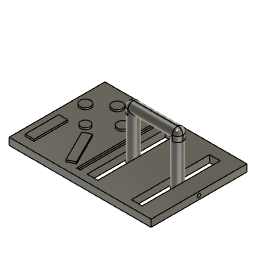
hardware final cad (Autodesk Fusion 360 design; units mm, degrees)
Autodesk Fusion 360 part; units mm, degrees
sketch "Sketch1" plane through (0, 0, 0) normal (0, 0, 1) x (1, 0, 0)
  line L0 (-8, -1) -> (1.5, -1)
  line L1 (1.5, -1) -> (1.5, -3.5)
  line L2 (1.5, -3.5) -> (-8, -3.5)
  line L3 (-8, -3.5) -> (-8, -1)
  line L4 (-11, 8) -> (-8, 8)
  line L5 (-8, 8) -> (-8, -14)
  line L6 (-8, -14) -> (-11, -14)
  line L7 (-11, -14) -> (-11, 8)
  line L8 (1.5, 8) -> (4.5, 8)
  line L9 (4.5, 8) -> (4.5, -14)
  line L10 (4.5, -14) -> (1.5, -14)
  line L11 (1.5, -14) -> (1.5, 8)
  line L12 (-19.5, -4) -> (-15, -13)
  line L13 (-15, -13) -> (-17, -14)
  line L14 (-17, -14) -> (-21.4999, -5.0003)
  line L15 (-19.5, -4) -> (-21.4999, -5.0003)
  line L16 (-29, -4) -> (-26.5, -4)
  line L17 (-26.5, -4) -> (-26.5, -13.5)
  line L18 (-26.5, -13.5) -> (-29, -13.5)
  line L19 (-29, -13.5) -> (-29, -4)
  circle A0 centre (-23, 6.5) radius 1.5
  circle A1 centre (-28, 2.5) radius 1.5
  circle A2 centre (-23, -2.5) radius 1.3194
  circle A3 centre (-17.5, 2.5) radius 1.5
  dimension "d1" = 10.062
  constraint horizontal L0
  constraint vertical L1
  constraint horizontal L2
  constraint vertical L3
  constraint horizontal L4
  constraint vertical L5
  constraint horizontal L6
  constraint vertical L7
  constraint horizontal L8
  constraint vertical L9
  constraint horizontal L10
  constraint vertical L11
  constraint perpendicular L12 L13
  constraint perpendicular L13 L14
  constraint horizontal L16
  constraint vertical L17
  constraint horizontal L18
  constraint vertical L19
  measures "d1" distance of L13.end L14.end
extrude "Extrude1" add sketch "Sketch1" along normal blind 1 makes body 1 at (-18.6666, -7.3334, 0) makes body 2 at (-23.2291, -1.2007, 0.6667) makes body 3 at (-16.0019, 2.4252, 0.6667) makes body 4 at (-28.1667, -7.1667, 0) makes body 5 at (-26.5019, 2.4252, 0.6667) makes body 6 at (-21.5019, 6.4252, 0.6667) makes body 7 at (-10, -3.1667, 0)
sketch "Sketch2" plane through (0, 0, 0) normal (0, 0, 1) x (1, 0, 0)
  line L0 (-31, 11) -> (9, 11)
  line L1 (9, 11) -> (9, -16)
  line L2 (9, -16) -> (-31, -16)
  line L3 (-31, -16) -> (-31, 11)
  constraint horizontal L0
  constraint vertical L1
  constraint horizontal L2
  constraint vertical L3
extrude "Extrude2" add sketch "Sketch2" against normal blind 1 separate body makes body 8
sketch "Sketch3" plane through (0, 0, 0) normal (0, 0, 1) x (-1, 0, 0)
  line L0 (31, 16) -> (-9, 16)
  line L1 (-9, 16) -> (-9, -11)
  line L2 (-9, -11) -> (31, -11)
  line L3 (31, -11) -> (31, 16)
  line L4 (13, -8) -> (12, -8)
  line L5 (12, -8) -> (12, 14.5)
  line L6 (12, 14.5) -> (13, 14.5)
  line L7 (13, 14.5) -> (13, -8)
  constraint horizontal L4
  constraint vertical L5
  constraint horizontal L6
  constraint vertical L7
extrude "Extrude3" cut 6 faces at (-18.6666, -7.3334, 1) (-23.361, -1.9445, 1) (-28.1667, -7.1667, 1) (-27.6335, 2.5453, 1) (-22.6335, 6.5453, 1) (-17.1335, 2.5453, 1) along direction (0, 0, -1) blind 1.5 on bodies 1 2 3 4 5 6 bodies 8
sketch "Sketch4" plane through (0, 0, 1) normal (0, 0, 1) x (-1, 0, 0)
  line L0 (-1.5, 14) -> (-4.5, 14)
  line L1 (-4.5, 14) -> (-4.5, -8)
  line L2 (-4.5, -8) -> (-1.5, -8)
  line L3 (-1.5, -8) -> (-1.5, 1)
  line L4 (-1.5, 1) -> (8, 1)
  line L5 (8, 1) -> (8, -8)
  line L6 (8, -8) -> (11, -8)
  line L7 (11, -8) -> (11, 14)
  line L8 (11, 14) -> (8, 14)
  line L9 (8, 14) -> (8, 3.5)
  line L10 (8, 3.5) -> (-1.5, 3.5)
  line L11 (-1.5, 3.5) -> (-1.5, 14)
  line L12 (8, 1) -> (-1.5, 1)
  line L13 (-1.5, 1) -> (-1.5, 3.5)
  line L14 (-1.5, 3.5) -> (8, 3.5)
  line L15 (8, 3.5) -> (8, 1)
  constraint horizontal L12
  constraint vertical L13
  constraint horizontal L14
  constraint vertical L15
  constraint coincident L10.end L11.start
  constraint coincident L4.end L5.start
extrude "Extrude4" cut sketch "Sketch4" against normal blind 2 contours L0 L1 L2 L3 L11 L13 | L5 L6 L7 L8 L9 L15 bodies 7 8
extrude "Extrude5" cut 1 faces at (-4.8333, -1.8333, 1) along direction (0, 0, -1) blind 1.5 on bodies 7 bodies 7 8
sketch "Sketch5" plane through (0, 0, 0) normal (0, 0, 1) x (-1, 0, 0)
  line L0 (8, 1) -> (-1.5, 1)
  line L1 (-1.5, 1) -> (-1.5, 3.5)
  line L2 (-1.5, 3.5) -> (8, 3.5)
  line L3 (8, 3.5) -> (8, 1)
  constraint horizontal L0
  constraint vertical L1
  constraint horizontal L2
  constraint vertical L3
extrude "Extrude6" add sketch "Sketch5" against normal blind 0.5 bodies 7 8
sketch "Sketch6" plane through (0, 0, 0) normal (0, 0, 1) x (1, 0, 0)
  circle A0 centre (-9.5, -2.5) radius 1.5
  circle A1 centre (3, -2.5) radius 1.5
extrude "Extrude8" add sketch "Sketch6" along normal blind 10 separate body makes body 9 at (-8.0019, -2.5748, 6.6667) makes body 10 at (4.4981, -2.5748, 6.6667)
sketch "Sketch7" plane through (0, 0, 10) normal (0, 0, 1) x (-1, 0, 0)
  circle A0 centre (-3, 2.5) radius 1.5
  line L0 (11, 1) -> (-4.5, 1)
  line L1 (-4.5, 1) -> (-4.5, 4)
  line L2 (-4.5, 4) -> (11, 4)
  line L3 (11, 4) -> (11, 1)
  constraint horizontal L0
  constraint vertical L1
  constraint horizontal L2
  constraint vertical L3
extrude "Extrude9" add sketch "Sketch7" along normal blind 3 bodies 9 10
fillet "Fillet1" radius 1.5 10 edges at (4.5, -2.5, 13) (4.5, -4, 11.5) (-3.25, -4, 13) (-11, -4, 11.5) (-3.25, -4, 10) (-11, -2.5, 13) (-11, -1, 11.5) (-3.25, -1, 13) (-3.25, -1, 10) (4.5, -1, 11.5) on bodies 9
sketch "Sketch8" plane through (0, 0, 0) normal (0, 0, 1) x (-1, 0, 0)
  line L0 (-1.5, 14) -> (-1.5, -8)
  line L1 (-1.5, -8) -> (-4.5, -8)
  line L2 (-4.5, -8) -> (-4.5, 14)
  line L3 (-4.5, 14) -> (-1.5, 14)
  line L4 (31, 16) -> (-9, 16)
  line L5 (-9, 16) -> (-9, -11)
  line L6 (-9, -11) -> (31, -11)
  line L7 (31, -11) -> (31, 16)
  circle A0 centre (17.5, -2.5) radius 1.5
  circle A1 centre (28, -2.5) radius 1.5
  circle A2 centre (23, 2.5) radius 1.3194
  line L8 (21.4999, 5.0003) -> (19.5, 4)
  line L9 (19.5, 4) -> (15, 13)
  line L10 (15, 13) -> (17, 14)
  line L11 (17, 14) -> (21.4999, 5.0003)
  line L12 (26.5, 4) -> (26.5, 13.5)
  line L13 (26.5, 13.5) -> (29, 13.5)
  line L14 (29, 13.5) -> (29, 4)
  line L15 (29, 4) -> (26.5, 4)
  circle A3 centre (23, -6.5) radius 1.5
  line L16 (8, -8) -> (8, 14)
  line L17 (8, 14) -> (11, 14)
  line L18 (11, 14) -> (11, -8)
  line L19 (11, -8) -> (8, -8)
  line L20 (8, 1) -> (-1.5, 1)
  line L21 (-1.5, 1) -> (-1.5, 4)
  line L22 (-1.5, 4) -> (8, 4)
  line L23 (8, 4) -> (8, 1)
  constraint horizontal L20
  constraint vertical L21
  constraint horizontal L22
  constraint vertical L23
  constraint coincident L0 L21.end
  constraint coincident L16 L20.start
extrude "Extrude10" add 1 faces at (-24.3333, 1, -1) along direction (0, 0, -1) blind 1 on bodies 7 bodies 7
move_body "Move1" bodies 9 to x (1, 0, 0) y (0, 1, 0) z (0, 0, 1) at (0, 0, 3)
extrude "Extrude11" add 2 faces at (3.4778, -2.6474, 3) (-8.9949, -2.7169, 3) along direction (0, 0, -1) blind 2 on bodies 9 bodies 9
move_body "Move2" bodies 9 to x (1, 0, 0) y (0, 1, 0) z (0, 0, 1) at (0, 0, -3)
sketch "Sketch9" plane through (9, 0, 0) normal (1, 0, 0) x (0, 1, 0)
  line L0 (11, 0) -> (-16, 0)
  line L1 (-16, 0) -> (-16, -2)
  line L2 (-16, -2) -> (11, -2)
  line L3 (11, -2) -> (11, 0)
  circle A0 centre (-2.5, -1) radius 0.5
extrude "Extrude12" cut sketch "Sketch9" against normal blind 22 contours A0 bodies 7 9
extrude "Extrude13" add 1 faces at (-13, -2.6803, -1.0054) along direction (1, 0, 0) blind 22 separate body on bodies 7 makes body 11
sketch "Sketch10" plane through (0, 0, 0) normal (0, 0, 1) x (-1, 0, 0)
  line L0 (-1.5, 14) -> (-1.5, -8)
  line L1 (-1.5, -8) -> (-4.5, -8)
  line L2 (-4.5, -8) -> (-4.5, 14)
  line L3 (-4.5, 14) -> (-1.5, 14)
  line L4 (31, 16) -> (-9, 16)
  line L5 (-9, 16) -> (-9, -11)
  line L6 (-9, -11) -> (31, -11)
  line L7 (31, -11) -> (31, 16)
  circle A0 centre (17.5, -2.5) radius 1.5
  circle A1 centre (28, -2.5) radius 1.5
  circle A2 centre (23, 2.5) radius 1.3194
  line L8 (21.4999, 5.0003) -> (19.5, 4)
  line L9 (19.5, 4) -> (15, 13)
  line L10 (15, 13) -> (17, 14)
  line L11 (17, 14) -> (21.4999, 5.0003)
  line L12 (26.5, 4) -> (26.5, 13.5)
  line L13 (26.5, 13.5) -> (29, 13.5)
  line L14 (29, 13.5) -> (29, 4)
  line L15 (29, 4) -> (26.5, 4)
  circle A3 centre (23, -6.5) radius 1.5
  line L16 (8, -8) -> (8, 14)
  line L17 (8, 14) -> (11, 14)
  line L18 (11, 14) -> (11, -8)
  line L19 (11, -8) -> (8, -8)
  line L20 (14, -8) -> (13, -8)
  line L21 (13, -8) -> (13, 14)
  line L22 (13, 14) -> (14, 14)
  line L23 (14, 14) -> (14, -8)
  constraint horizontal L20
  constraint vertical L21
  constraint horizontal L22
  constraint vertical L23
extrude "Extrude14" cut sketch "Sketch10" against normal blind 0.5 contours L20 L21 L22 L23 bodies 7
move_body "Move3" bodies 1 5 6 2 3 4 to x (1, 0, 0) y (0, 1, 0) z (0, 0, 1) at (0, 0, -0.5)
